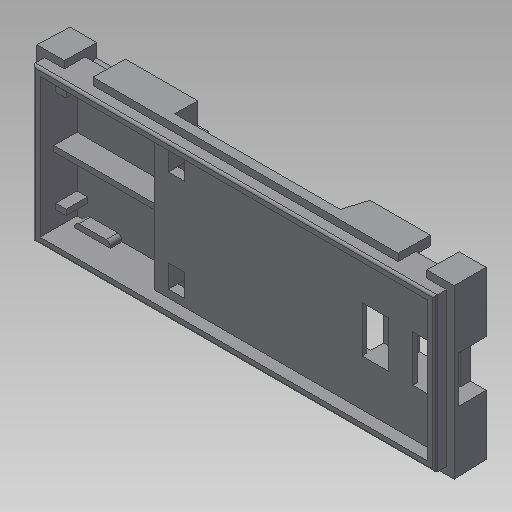
# Autodesk Inventor part: D2MG bottom
Saved by Autodesk Inventor 2018 (Build 220112000, 112)
## iProperties
Created: 2015-02-09
Part Number: D2MG bottom
Material: Типовые
Document SubType Name: Modeling
Designer: Abbath
Density: 1 g/cm^3
Appearance: По умолчанию
Mass: 9.33174 g
Surface Area: 109.957 cm^2
Volume: 9.33174 cm^3
Author: Abbath
Autodesk Inventor part; units mm, degrees
sketch "Эскиз2" plane through (0, 0, 0) normal (0, 1, 0) x (-1, 0, 0)
  line L0 (45.1, 0) -> (-45.1, 0)
  line L1 (-45.1, 0) -> (-44.9342, -9.5)
  line L2 (-44.9342, -9.5) -> (44.9342, -9.5)
  line L3 (44.9342, -9.5) -> (45.1, 0)
  line L4 (-45.1, 0) -> (-45.1, -33.7167) construction
  line L5 (45.1, 0) -> (45.1, -29.7578) construction
  point P0 (0, 0)
  point P1 (0, 0)
  dimension "d4" = 9.5
  dimension "d5" = 90.2
  dimension "d6" = 1
  dimension "d7" = 1
  constraints: 12 end point, 2 vertical, 1 coincident, 1 horizontal, 1 midpoint, 1 parallel
  measures "d4" distance between parallel lines of L2 L0
  measures "d5" distance of L0.start L0.end
  measures "d6" angle of L4 L1
  measures "d7" angle of L3 L5
sketch "Эскиз3" plane through (0, 0, 0) normal (1, 0, 0) x (0, 1, 0)
  line L0 (-18.15, 0) -> (18.15, 0)
  line L1 (18.15, 0) -> (17.9842, -9.5)
  line L2 (17.9842, -9.5) -> (-17.9842, -9.5)
  line L3 (-17.9842, -9.5) -> (-18.15, 0)
  line L4 (18.15, 0) -> (18.15, -16.3653) construction
  line L5 (-18.15, 0) -> (-18.15, -16.3653) construction
  point P0 (0, 0)
  point P1 (0, 0)
  point P2 (0, -9.5)
  point P3 (0, 0)
  point P4 (0, -9.5)
  dimension "d8" = 1
  dimension "d9" = 1
  dimension "d10" = 36.3
  constraints: 12 end point, 2 coincident, 2 midpoint, 2 vertical, 1 horizontal, 1 parallel
  measures "d8" angle of L5 L3
  measures "d9" angle of L4 L1
  measures "d10" distance of L0.start L0.end
ref_plane "РабПлоскость1" through (-45.1, 0, 0) normal (0, 0, 1) x (1, 0, 0)
sketch "Эскиз4" plane through (-45.1, 0, 0) normal (0, 0, 1) x (1, 0, 0)
  line L0 (0, 18.15) -> (90.2, 18.15)
  line L1 (90.2, 18.15) -> (90.2, -18.15)
  line L2 (90.2, -18.15) -> (0, -18.15)
  line L3 (0, -18.15) -> (0, 18.15)
  point P0 (45.1, 0)
  point P1 (0, 0)
  point P2 (45.1, 18.15)
  point P3 (90.2, 0)
  point P4 (45.1, -18.15)
  constraints: 8 end point, 4 midpoint, 2 parallel, 1 horizontal, 1 perpendicular
ref_plane "РабПлоскость2" through (44.9342, 0, -9.5) normal (0, 0, 1) x (-1, 0, 0)
sketch "Эскиз5" plane through (44.9342, 0, -9.5) normal (0, 0, 1) x (-1, 0, 0)
  line L0 (89.8684, -17.9842) -> (0, -17.9842)
  line L1 (0, -17.9842) -> (0, 17.9842)
  line L2 (0, 17.9842) -> (89.8684, 17.9842)
  line L3 (89.8684, 17.9842) -> (89.8684, -17.9842)
  point P0 (44.9342, 0)
  point P1 (89.8684, 0)
  point P2 (44.9342, -17.9842)
  point P3 (0, 0)
  point P4 (44.9342, 17.9842)
  constraints: 8 end point, 4 midpoint, 2 parallel, 1 horizontal, 1 perpendicular
loft "Лофт1" add profiles "Эскиз5", "Эскиз4"
sketch "Эскиз6" plane through (-45.1, 18.15, 0) normal (0, 0, 1) x (1, 0, 0)
  line L0 (1.7, -34.7) -> (88.5, -34.7)
  line L1 (88.5, -34.7) -> (88.5, -1.6)
  line L2 (88.5, -1.6) -> (1.7, -1.6)
  line L3 (1.7, -1.6) -> (1.7, -34.7)
  line L4 (0, -36.3) -> (0, 0) construction
  line L5 (90.2, -36.3) -> (0, -36.3) construction
  line L6 (90.2, 0) -> (90.2, -36.3) construction
  line L7 (0, 0) -> (90.2, 0) construction
  line L8 (-1, -37.3) -> (91.2, -37.3)
  line L9 (91.2, -37.3) -> (91.2, 1)
  line L10 (91.2, 1) -> (-1, 1)
  line L11 (-1, 1) -> (-1, -37.3)
  point P0 (45.1, -18.15)
  point P1 (45.1, -1.6)
  point P2 (1.7, -18.15)
  dimension "d21" = 86.8
  dimension "d22" = 1.7
  dimension "d23" = 1.7
  dimension "d24" = 33.1
  dimension "d25" = 1.6
  dimension "d26" = 1.6
  dimension "d27" = 1
  dimension "d28" = 1
  dimension "d29" = 1
  dimension "d30" = 1
  constraints: 16 end point, 4 parallel, 2 horizontal, 2 midpoint, 2 perpendicular, 1 horizontal alignment, 1 vertical alignment
  measures "d21" distance between parallel lines of L1 L3
  measures "d22" distance between parallel lines of L3 L4
  measures "d23" distance between parallel lines of L6 L1
  measures "d24" distance between parallel lines of L2 L0
  measures "d25" distance between parallel lines of L0 L5
  measures "d26" distance between parallel lines of L7 L2
  measures "d27" distance between parallel lines of L4 L11
  measures "d28" distance between parallel lines of L10 L7
  measures "d29" distance between parallel lines of L9 L6
  measures "d30" distance between parallel lines of L8 L5
extrude "Выдавливание2" cut sketch "Эскиз6" against normal blind 2.5
sketch "Эскиз7" plane through (-43.4, 16.55, 0) normal (0, 0, 1) x (1, 0, 0)
  line L0 (1.5, -31.6) -> (85.3, -31.6)
  line L1 (85.3, -31.6) -> (85.3, -1.5)
  line L2 (85.3, -1.5) -> (1.5, -1.5)
  line L3 (1.5, -1.5) -> (1.5, -31.6)
  line L4 (86.8, -33.1) -> (86.8, 0) construction
  line L5 (86.8, 0) -> (0, 0) construction
  line L6 (0, 0) -> (0, -33.1) construction
  line L7 (0, -33.1) -> (86.8, -33.1) construction
  point P0 (43.4, -16.55)
  dimension "d33" = 1.5
  dimension "d34" = 1.5
  dimension "d35" = 1.5
  dimension "d36" = 1.5
  constraints: 8 end point, 2 parallel, 1 horizontal, 1 perpendicular
  measures "d33" distance between parallel lines of L3 L6
  measures "d34" distance between parallel lines of L2 L5
  measures "d35" distance between parallel lines of L1 L4
  measures "d36" distance between parallel lines of L0 L7
extrude "Выдавливание3" cut sketch "Эскиз7" against normal blind 2.5
sketch "Эскиз8" plane through (-43.4, 16.55, -2.5) normal (0, 0, 1) x (1, 0, 0)
  line L0 (1.5, -1.5) -> (23.8, -1.5)
  line L1 (23.8, -1.5) -> (23.8, -31.6)
  line L2 (23.8, -31.6) -> (1.5, -31.6)
  line L3 (1.5, -31.6) -> (1.5, -1.5)
  line L4 (85.3, -31.6) -> (1.5, -31.6) construction
  line L5 (85.3, -1.5) -> (85.3, -31.6) construction
  line L6 (1.5, -1.5) -> (85.3, -1.5) construction
  line L7 (1.5, -31.6) -> (1.5, -1.5) construction
  point P0 (43.4, -16.55)
  dimension "d39" = 22.3
  constraints: 8 end point, 3 collinear, 2 parallel, 1 horizontal, 1 perpendicular
  measures "d39" distance between parallel lines of L1 L3
extrude "Выдавливание4" cut sketch "Эскиз8" against normal blind 5.5
sketch "Эскиз9" plane through (0, 0, 0) normal (0, 1, 0) x (-1, 0, 0)
  line L0 (19.6, -8) -> (41.9, -8)
  line L1 (41.9, -8) -> (41.9, -3)
  line L2 (41.9, -3) -> (19.6, -3)
  line L3 (19.6, -3) -> (19.6, -8)
  line L4 (19.6, -2.5) -> (19.6, -8) construction
  line L5 (19.6, -8) -> (41.9, -8) construction
  line L6 (41.9, 0) -> (41.9, -8) construction
  line L7 (-44.9342, -9.5) -> (44.9342, -9.5) construction
  line L8 (-41.9, -2.5) -> (19.6, -2.5) construction
  point P0 (0, 0)
  dimension "d43" = 0.5
  constraints: 8 end point, 3 collinear, 2 parallel, 1 horizontal, 1 perpendicular
  measures "d43" distance between parallel lines of L2 L8
extrude "Выдавливание5" add sketch "Эскиз9" along normal mid plane 1.2
sketch "Эскиз10" plane through (-43.4, 16.55, 0) normal (0, 0, 1) x (1, 0, 0)
  line L0 (4.25, -33.1) -> (10.45, -33.1)
  line L1 (10.45, -33.1) -> (10.45, -35.6564)
  line L2 (10.45, -35.6564) -> (4.25, -35.6564)
  line L3 (4.25, -35.6564) -> (4.25, -33.1)
  line L4 (4.25, 2.5564) -> (10.45, 2.5564)
  line L5 (10.45, 2.5564) -> (10.45, 0)
  line L6 (10.45, 0) -> (4.25, 0)
  line L7 (4.25, 0) -> (4.25, 2.5564)
  line L8 (76.35, 0) -> (82.55, 0)
  line L9 (82.55, 0) -> (82.55, 2.5564)
  line L10 (82.55, 2.5564) -> (76.35, 2.5564)
  line L11 (76.35, 2.5564) -> (76.35, 0)
  line L12 (76.35, -33.1) -> (82.55, -33.1)
  line L13 (82.55, -33.1) -> (82.55, -35.6564)
  line L14 (82.55, -35.6564) -> (76.35, -35.6564)
  line L15 (76.35, -35.6564) -> (76.35, -33.1)
  line L16 (7.35, -51.2865) -> (7.35, 35.2838) construction
  line L17 (79.45, -51.2865) -> (79.45, 29.244) construction
  line L18 (-1.6564, 1.5564) -> (88.4564, 1.5564) construction
  line L19 (-1.6564, -34.6564) -> (-1.6564, 1.5564) construction
  line L20 (88.4564, -34.6564) -> (-1.6564, -34.6564) construction
  line L21 (88.4564, 1.5564) -> (88.4564, -34.6564) construction
  line L22 (86.8, -33.1) -> (86.8, 0) construction
  line L23 (0, -33.1) -> (86.8, -33.1) construction
  line L24 (0, 0) -> (0, -33.1) construction
  line L25 (86.8, 0) -> (0, 0) construction
  line L26 (86.8, 0) -> (0, 0) construction
  point P0 (43.4, -16.55)
  point P1 (7.35, 2.5564)
  point P2 (7.35, -35.6564)
  point P3 (79.45, -35.6564)
  point P4 (79.45, 0)
  dimension "d46" = 72.1
  dimension "d47" = 36.05
  dimension "d48" = 6.2
  dimension "d49" = 1
  constraints: 36 end point, 8 parallel, 6 point on line, 5 collinear, 4 horizontal, 4 midpoint, 4 perpendicular, 3 equal length, 2 vertical
  measures "d46" distance between parallel lines of L17 L16
  measures "d47" distance from line of point (43.4, -16.55) L16
  measures "d48" distance between parallel lines of L5 L7
  measures "d49" distance between parallel lines of L10 L18
extrude "Выдавливание6" cut sketch "Эскиз10" against normal through all
sketch "Эскиз11" plane through (-43.4, 16.55, -8) normal (0, 0, 1) x (1, 0, 0)
  line L0 (1.5, -31.6) -> (1.5, -1.5) construction
  line L1 (85.3, -31.6) -> (1.5, -31.6) construction
  line L2 (1.5, -1.5) -> (85.3, -1.5) construction
  line L3 (3.5, -31.6) -> (11.2, -31.6)
  line L4 (3.5, -31.6) -> (3.5, -31.3)
  line L5 (4.4, -30.4) -> (10.3, -30.4)
  line L6 (11.2, -31.3) -> (11.2, -31.6)
  line L7 (3.5, -1.5) -> (11.2, -1.5)
  line L8 (11.2, -1.5) -> (11.2, -1.8)
  line L9 (10.3, -2.7) -> (4.4, -2.7)
  line L10 (3.5, -1.8) -> (3.5, -1.5)
  arc A0 (3.5, -1.8) -> (4.4, -2.7) centre (4.4, -1.8) ccw
  arc A1 (10.3, -2.7) -> (11.2, -1.8) centre (10.3, -1.8) ccw
  arc A2 (4.4, -30.4) -> (3.5, -31.3) centre (4.4, -31.3) ccw
  arc A3 (11.2, -31.3) -> (10.3, -30.4) centre (10.3, -31.3) ccw
  line L11 (1.5, -28.15) -> (3.7436, -28.15)
  line L12 (3.7436, -28.15) -> (3.7436, -26.95)
  line L13 (3.7436, -26.95) -> (1.5, -26.95)
  line L14 (1.5, -26.95) -> (1.5, -28.15)
  line L15 (1.5, -6.15) -> (3.7436, -6.15)
  line L16 (3.7436, -6.15) -> (3.7436, -4.95)
  line L17 (3.7436, -4.95) -> (1.5, -4.95)
  line L18 (1.5, -4.95) -> (1.5, -6.15)
  line L19 (4.25, -33.1) -> (4.25, -34.5342) projected
  line L20 (10.45, -34.5342) -> (10.45, -33.1) projected
  line L21 (-1.6564, -34.6564) -> (-1.6564, 1.5564) projected
  point P0 (43.4, -16.55)
  dimension "d52" = 7.7
  dimension "d53" = 0.75
  dimension "d54" = 0.75
  dimension "d55" = 1.2
  dimension "d56" = 0.9
  dimension "d57" = 20.8
  dimension "d58" = 10.4
  dimension "d59" = 23.2
  dimension "d72" = 5.4
  constraints: 32 end point, 8 point on circle, 8 tangent, 7 perpendicular, 5 collinear, 4 centre point, 4 horizontal, 4 parallel, 3 equal radius, 2 equal length, 2 point on line, 1 vertical
  measures "d52" distance between parallel lines of L6 L4
  measures "d53" distance between parallel lines of L19 L4
  measures "d54" distance between parallel lines of L6 L20
  measures "d55" distance between parallel lines of L5 L3
  measures "d56" radius of A2
  measures "d57" distance between parallel lines of L15 L13
  measures "d58" distance from line of point (43.4, -16.55) L13
  measures "d59" distance between parallel lines of L17 L11
  measures "d72" distance between parallel lines of L16 L21
extrude "Выдавливание7" add sketch "Эскиз11" along normal blind 4.6 contours L14 L13 L12 L11 | L18 L17 L16 L15
fillet "Сопряжение1" radius 0.5 4 edges at (0, -16.55, 0) (43.4, 0, 0) (0, 16.55, 0) (-43.4, 0, 0)
sketch "Эскиз12" plane through (-32.95, -16.55, -2.5) normal (0, -1, 0) x (1, 0, 0)
  line L0 (-6.2, -7) -> (-6.2, 0) construction
  line L1 (0, 0) -> (0, -7) construction
  line L2 (65.9, -7) -> (65.9, 0) construction
  line L3 (72.1, 0) -> (72.1, -7) construction
  line L4 (-6.2, -4.5) -> (0, -4.5)
  line L5 (0, -4.5) -> (0, -8)
  line L6 (0, -8) -> (-6.2, -8)
  line L7 (-6.2, -8) -> (-6.2, -4.5)
  line L8 (65.9, -4.5) -> (72.1, -4.5)
  line L9 (72.1, -4.5) -> (72.1, -8)
  line L10 (72.1, -8) -> (65.9, -8)
  line L11 (65.9, -8) -> (65.9, -4.5)
  line L12 (65.9, 0) -> (0, 0) construction
  line L13 (0, -7) -> (65.9, -7) construction
  point P0 (32.95, 2.5)
  dimension "d64" = 4.5
  dimension "d65" = 1
  constraints: 16 end point, 4 collinear, 4 parallel, 2 horizontal, 2 perpendicular, 2 point on line
  measures "d64" distance between parallel lines of L4 L12
  measures "d65" distance between parallel lines of L6 L13
extrude "Выдавливание8" cut sketch "Эскиз12" against normal up to surface (1.5 mm away)
sketch "Эскиз13" plane through (-32.95, 16.55, -2.5) normal (0, 1, 0) x (1, 0, 0)
  line L0 (-6.2, 8) -> (-6.2, 4.5) projected
  line L1 (0, 8) -> (-6.2, 8) projected
  line L2 (0, 4.5) -> (0, 8) projected
  line L3 (-6.2, 4.5) -> (0, 4.5) projected
  line L4 (65.9, 4.5) -> (72.1, 4.5) projected
  line L5 (72.1, 4.5) -> (72.1, 8) projected
  line L6 (65.9, 8) -> (65.9, 4.5) projected
  line L7 (72.1, 8) -> (65.9, 8) projected
  point P0 (32.95, -2.5)
extrude "Выдавливание9" cut sketch "Эскиз13" against normal up to surface (1.5 mm away)
extrude "Выдавливание10" add sketch "Эскиз11" along normal blind 2.5 contours L4 A2 L5 A3 L6 L3 | L7 L8 A1 L9 A0 L10
ref_plane "РабПлоскость3" through (-32.95, 0, -2.5) normal (0, -1, 0) x (1, 0, 0)
ref_plane "РабПлоскость4" through (0, -16.55, -2.5) normal (1, 0, 0) x (0, 0, -1)
sketch "Эскиз14" plane through (44.9342, -17.9842, -9.5) normal (0, 0, -1) x (-1, 0, 0)
  line L0 (2, 2) -> (62.2684, 2)
  line L1 (62.2684, 2) -> (62.2684, 33.9684)
  line L2 (62.2684, 33.9684) -> (2, 33.9684)
  line L3 (2, 33.9684) -> (2, 2)
  line L4 (89.8684, 0) -> (89.8684, 35.9684) construction
  line L5 (11.9842, 0) -> (77.8842, 0) construction
  line L6 (77.8842, 35.9684) -> (11.9842, 35.9684) construction
  line L7 (0, 35.9684) -> (0, 0) construction
  line L8 (5.7842, 35.9684) -> (0, 35.9684) projected
  point P0 (44.9342, 17.9842)
  dimension "d73" = 27.6
  dimension "d74" = 2
  dimension "d75" = 2
  dimension "d76" = 2
  constraints: 8 end point, 2 parallel, 1 horizontal, 1 perpendicular
  measures "d73" distance between parallel lines of L1 L4
  measures "d74" distance between parallel lines of L3 L7
  measures "d75" distance between parallel lines of L2 L8
  measures "d76" distance between parallel lines of L0 L5
extrude "Выдавливание11" cut sketch "Эскиз14" against normal blind 5
sketch "Эскиз15" plane through (0, 0, 0) normal (0, 1, 0) x (-1, 0, 0)
  line L0 (17.3342, -9.5) -> (17.3342, -4.5) construction
  line L1 (-42.9342, -4.5) -> (17.3342, -4.5) construction
  line L2 (17.3342, -9.5) -> (17.3342, -4.5)
  line L3 (17.3342, -4.5) -> (-18.4658, -4.5)
  line L4 (-18.4658, -4.5) -> (-19.8658, -9.5)
  line L5 (-19.8658, -9.5) -> (17.3342, -9.5)
  line L6 (-32.95, -9.5) -> (17.3342, -9.5) construction
  point P0 (0, 0)
  dimension "d79" = 35.8
  dimension "d80" = 37.2
  constraints: 8 end point, 3 collinear, 2 horizontal, 1 vertical
  measures "d79" distance from line of L3.end L0
  measures "d80" distance from line of L4.end L0
extrude "Выдавливание12" cut sketch "Эскиз15" along normal through all both and the other way through all
ref_plane "РабПлоскость5" through (44.9342, -17.9842, -3.5) normal (0, 0, -1) x (-1, 0, 0)
sketch "Эскиз16" plane through (44.9342, -17.9842, -3.5) normal (0, 0, -1) x (-1, 0, 0)
  line L0 (0, 35.9684) -> (0, 0) construction
  line L1 (62.2684, 35.9684) -> (62.2684, 0) construction
  line L2 (62.2684, -0.0873) -> (26.4684, -0.0873) construction
  line L3 (26.4684, 36.0556) -> (62.2684, 36.0556) construction
  line L4 (-5, 12.9842) -> (51.9905, 12.9842)
  line L5 (51.9905, 12.9842) -> (51.9905, 22.9842)
  line L6 (51.9905, 22.9842) -> (-5, 22.9842)
  line L7 (-5, 22.9842) -> (-5, 12.9842)
  line L8 (89.9905, -0.1222) -> (89.9905, 36.0905) construction
  point P0 (44.9342, 17.9842)
  point P1 (51.9905, 17.9842)
  dimension "d84" = 10
  dimension "d85" = 5
  dimension "d86" = 38
  constraints: 8 end point, 2 parallel, 1 horizontal, 1 horizontal alignment, 1 midpoint, 1 perpendicular
  measures "d84" distance between parallel lines of L6 L4
  measures "d85" distance between parallel lines of L7 L0
  measures "d86" distance between parallel lines of L5 L8
extrude "Выдавливание13" cut sketch "Эскиз16" along normal through all
sketch "Эскиз17" plane through (44.9342, -17.9842, -3.5) normal (0, 0, -1) x (-1, 0, 0)
  line L0 (-0.1047, 12.9842) -> (-0.1047, 22.9842) construction
  line L1 (-0.1047, 12.9842) -> (51.9905, 12.9842) construction
  line L2 (51.9905, 12.9842) -> (51.9905, 22.9842) construction
  line L3 (51.9905, 22.9842) -> (-0.1047, 22.9842) construction
  line L4 (13.9842, 12.9842) -> (19.7842, 12.9842)
  line L5 (19.7842, 12.9842) -> (19.7842, 22.9842)
  line L6 (19.7842, 22.9842) -> (13.9842, 22.9842)
  line L7 (13.9842, 22.9842) -> (13.9842, 12.9842)
  line L8 (3.0342, 12.9842) -> (8.8342, 12.9842)
  line L9 (8.8342, 12.9842) -> (8.8342, 22.9842)
  line L10 (8.8342, 22.9842) -> (3.0342, 22.9842)
  line L11 (3.0342, 22.9842) -> (3.0342, 12.9842)
  line L12 (3.0342, 33.0342) -> (3.0342, 2.9342) construction
  point P0 (44.9342, 17.9842)
  dimension "d89" = 5.8
  dimension "d90" = 5.15
  constraints: 16 end point, 6 collinear, 4 parallel, 2 horizontal, 2 perpendicular
  measures "d89" distance between parallel lines of L9 L12
  measures "d90" distance between parallel lines of L7 L9
extrude "Выдавливание14" cut sketch "Эскиз17" against normal through all
sketch "Эскиз18" plane through (0, 0, 0) normal (0, 1, 0) x (-1, 0, 0)
  line L0 (-32.95, -9.5) -> (-32.95, -2.5) construction
  line L1 (-39.15, -2.5) -> (-39.15, -9.5) construction
  line L2 (-42.9, 0) -> (42.9, 0) construction
  line L3 (-32.95, -6.3) -> (-39.15, -6.3)
  line L4 (-39.15, -6.3) -> (-39.15, -8)
  line L5 (-39.15, -8) -> (-32.95, -8)
  line L6 (-32.95, -8) -> (-32.95, -6.3)
  line L7 (-39.15, -7) -> (-32.95, -7) projected
  point P0 (0, 0)
  dimension "d93" = 1
  dimension "d94" = 6.3
  constraints: 8 end point, 2 collinear, 2 parallel, 1 horizontal, 1 perpendicular
  measures "d93" distance between parallel lines of L5 L7
  measures "d94" distance between parallel lines of L2 L3
extrude "Выдавливание15" cut sketch "Эскиз18" along normal through all both and the other way through all
sketch "Эскиз19" plane through (44.9342, -17.9842, -4.5) normal (0, 0, -1) x (-1, 0, 0)
  line L0 (11.9842, 1.4342) -> (5.7842, 1.4342) construction
  line L1 (5.7842, 34.5342) -> (11.9842, 34.5342) construction
  line L2 (4.4842, 1.4342) -> (13.2842, 1.4342)
  arc A0 (13.2842, 1.4342) -> (11.9842, 2.7342) centre (11.9842, 1.4342) ccw
  line L3 (11.9842, 2.7342) -> (5.7842, 2.7342)
  arc A1 (5.7842, 2.7342) -> (4.4842, 1.4342) centre (5.7842, 1.4342) ccw
  line L4 (4.4842, 34.5342) -> (13.2842, 34.5342)
  arc A2 (11.9842, 33.2342) -> (13.2842, 34.5342) centre (11.9842, 34.5342) ccw
  line L5 (11.9842, 33.2342) -> (5.7842, 33.2342)
  arc A3 (4.4842, 34.5342) -> (5.7842, 33.2342) centre (5.7842, 34.5342) ccw
  line L6 (5.7842, 36.0905) -> (5.7842, 34.5342) construction
  line L7 (11.9842, 34.5342) -> (11.9842, 36.0905) construction
  line L8 (5.7842, 1.4342) -> (5.7842, -0.1222) construction
  line L9 (11.9842, -0.1222) -> (11.9842, 1.4342) construction
  point P0 (44.9342, 17.9842)
  dimension "d97" = 1.3
  dimension "d98" = 1.3
  constraints: 8 end point, 8 point on circle, 8 point on line, 4 centre point, 4 horizontal, 4 vertical alignment, 2 collinear
  measures "d97" distance between parallel lines of L3 L2
  measures "d98" distance between parallel lines of L5 L4
extrude "Выдавливание16" add sketch "Эскиз19" along normal up to surface (1.8 mm away)
sketch "Эскиз20" plane through (44.9342, -17.9842, -4.5) normal (0, 0, -1) x (-1, 0, 0)
  line L0 (19.8778, 24.9842) -> (2, 24.9842)
  line L1 (2, 24.9842) -> (2, 22.9842)
  line L2 (2, 22.9842) -> (19.8778, 22.9842)
  line L3 (19.8778, 22.9842) -> (19.8778, 24.9842)
  line L4 (19.8778, 12.9842) -> (2, 12.9842)
  line L5 (2, 12.9842) -> (2, 10.9842)
  line L6 (2, 10.9842) -> (19.8778, 10.9842)
  line L7 (19.8778, 10.9842) -> (19.8778, 12.9842)
  line L8 (51.9905, 12.9842) -> (2, 12.9842) construction
  line L9 (2, 22.9842) -> (51.9905, 22.9842) construction
  line L10 (2, 22.9842) -> (2, 33.9684) construction
  line L11 (2, 2) -> (2, 12.9842) construction
  line L12 (-0.1222, 36.0905) -> (-0.1222, -0.1222) construction
  point P0 (44.9342, 17.9842)
  dimension "d101" = 14
  dimension "d102" = 20
  constraints: 16 end point, 6 collinear, 4 parallel, 2 horizontal, 2 perpendicular
  measures "d101" distance between parallel lines of L6 L0
  measures "d102" distance between parallel lines of L7 L12
extrude "Выдавливание17" add sketch "Эскиз20" along normal up to surface (5 mm away)
sketch "Эскиз21" plane through (0, 0, 0) normal (0, 1, 0) x (-1, 0, 0)
  line L0 (-44.9342, -9.5) -> (-45.0389, -3.5) construction
  line L1 (-25.0564, -9.5) -> (-44.9342, -9.5) construction
  line L2 (-25.0564, -4.5) -> (-25.0564, -9.5) construction
  line L3 (-25.0564, -7.3) -> (-30.5564, -7.3)
  line L4 (-30.5564, -7.3) -> (-30.5564, -9.5)
  line L5 (-30.5564, -9.5) -> (-25.0564, -9.5)
  line L6 (-25.0564, -9.5) -> (-25.0564, -7.3)
  line L7 (-36.4564, -7.3) -> (-41.5564, -7.3)
  line L8 (-41.5564, -7.3) -> (-41.5564, -9.5)
  line L9 (-41.5564, -9.5) -> (-36.4564, -9.5)
  line L10 (-36.4564, -9.5) -> (-36.4564, -7.3)
  point P0 (0, 0)
  dimension "d105" = 5.5
  dimension "d106" = 5.9
  dimension "d107" = 5.1
  dimension "d108" = 2.2
  constraints: 16 end point, 4 collinear, 4 parallel, 2 horizontal, 2 perpendicular
  measures "d105" distance between parallel lines of L4 L2
  measures "d106" distance between parallel lines of L10 L4
  measures "d107" distance between parallel lines of L8 L10
  measures "d108" distance between parallel lines of L3 L1
extrude "Выдавливание18" add sketch "Эскиз21" along normal up to surface (10 mm away) from surface at -5
sketch "Эскиз22" plane through (44.9342, -17.9842, -4.5) normal (0, 0, -1) x (-1, 0, 0)
  arc A0 (21.1278, 5.7778) -> (21.1278, 3.2778) centre (21.1278, 4.5278) ccw
  arc A1 (22.0278, 3.2778) -> (22.0278, 5.7778) centre (22.0278, 4.5278) ccw
  arc A2 (21.1278, 32.6905) -> (21.1278, 30.1905) centre (21.1278, 31.4405) ccw
  arc A3 (22.0278, 30.1905) -> (22.0278, 32.6905) centre (22.0278, 31.4405) ccw
  line L0 (21.1278, 3.2778) -> (22.0278, 3.2778)
  line L1 (21.1278, 5.7778) -> (22.0278, 5.7778)
  line L2 (21.1278, 30.1905) -> (22.0278, 30.1905)
  line L3 (21.1278, 32.6905) -> (22.0278, 32.6905)
  line L4 (19.8778, 3.5894) -> (19.8778, 6.2353) construction
  line L5 (23.2778, 3.5894) -> (23.2778, 5.4774) construction
  line L6 (11.9842, -0.1222) -> (77.8842, -0.1222) construction
  line L7 (77.8842, 36.0905) -> (11.9842, 36.0905) construction
  line L8 (-0.1222, 36.0905) -> (-0.1222, -0.1222) construction
  point P0 (44.9342, 17.9842)
  dimension "d111" = 3.4
  dimension "d112" = 2.5
  dimension "d113" = 5.9
  dimension "d114" = 5.9
  dimension "d115" = 23.4
  constraints: 12 end point, 10 tangent, 8 point on circle, 4 centre point, 4 horizontal, 2 vertical, 1 equal radius, 1 parallel, 1 vertical alignment
  measures "d111" distance between parallel lines of L5 L4
  measures "d112" distance between parallel lines of L1 L0
  measures "d113" distance between parallel lines of L2 L7
  measures "d114" distance between parallel lines of L1 L6
  measures "d115" distance between parallel lines of L5 L8
extrude "Выдавливание19" add sketch "Эскиз22" along normal blind 3
sketch "Эскиз23" plane through (44.9342, -17.9842, -4.5) normal (0, 0, -1) x (-1, 0, 0)
  line L0 (89.9905, -0.1222) -> (89.9905, 36.0905) construction
  line L1 (77.8842, 36.0905) -> (11.9842, 36.0905) construction
  line L2 (11.9842, -0.1222) -> (77.8842, -0.1222) construction
  line L3 (58.0905, 4.5778) -> (61.5905, 4.5778)
  line L4 (61.5905, 4.5778) -> (61.5905, 9.4842)
  line L5 (61.5905, 9.4842) -> (58.0905, 9.4842)
  line L6 (58.0905, 9.4842) -> (58.0905, 4.5778)
  line L7 (58.0905, 26.4842) -> (61.5905, 26.4842)
  line L8 (61.5905, 26.4842) -> (61.5905, 31.3905)
  line L9 (61.5905, 31.3905) -> (58.0905, 31.3905)
  line L10 (58.0905, 31.3905) -> (58.0905, 26.4842)
  point P0 (44.9342, 17.9842)
  dimension "d118" = 28.4
  dimension "d119" = 4.7
  dimension "d120" = 4.7
  dimension "d121" = 17
  dimension "d122" = 3.5
  constraints: 16 end point, 4 parallel, 3 collinear, 2 horizontal, 2 perpendicular
  measures "d118" distance between parallel lines of L8 L0
  measures "d119" distance between parallel lines of L9 L1
  measures "d120" distance between parallel lines of L3 L2
  measures "d121" distance between parallel lines of L7 L5
  measures "d122" distance between parallel lines of L4 L6
extrude "Выдавливание20" cut sketch "Эскиз23" against normal through all
ref_plane "РабПлоскость6" through (-16.6564, -10.9532, -4.5) normal (0, -1, 0) x (1, 0, 0)
sketch "Эскиз24" plane through (-16.6564, -10.9532, -4.5) normal (0, -1, 0) x (1, 0, 0)
  line L0 (0, 0) -> (-0.6778, 0)
  line L1 (-0.6778, 0) -> (-0.6778, -5)
  line L2 (-0.6778, -5) -> (1.6, -5)
  line L3 (1.6, -5) -> (1.6, -3)
  line L4 (1.6, -3) -> (0, -2.0762)
  line L5 (0, -2.0762) -> (0, 0)
  line L6 (35.1222, 0) -> (-0.6778, 0) construction
  line L7 (-0.6778, 0) -> (-0.6778, -5) construction
  line L8 (0, 0) -> (0, 2) construction
  line L9 (-16.2936, -5) -> (-0.6778, -5) construction
  line L10 (-28.2778, -5) -> (-28.4, 2) construction
  point P0 (16.6564, 4.5)
  dimension "d125" = 30
  dimension "d126" = 2
  dimension "d127" = 60
  constraints: 12 end point, 4 collinear, 3 vertical, 2 horizontal
  measures "d125" distance from line of L3 L10.end
  measures "d126" distance of L2.end L3.end
  measures "d127" angle of L4 L5
extrude "Выдавливание21" add sketch "Эскиз24" along normal up to surface (4.9064 mm away) from surface at -2.4532
ref_plane "РабПлоскость7" through (-16.6564, 10.9532, -4.5) normal (0, 1, 0) x (1, 0, 0)
sketch "Эскиз25" plane through (-16.6564, 10.9532, -4.5) normal (0, 1, 0) x (1, 0, 0)
  line L0 (0, 0) -> (0, 2.0762) projected
  line L1 (-0.6778, 0) -> (0, 0) projected
  line L2 (-0.6778, 5) -> (-0.6778, 0) projected
  line L3 (1.6, 5) -> (-0.6778, 5) projected
  line L4 (1.6, 3) -> (1.6, 5) projected
  line L5 (0, 2.0762) -> (1.6, 3) projected
  point P0 (16.6564, -4.5)
extrude "Выдавливание22" add sketch "Эскиз25" against normal up to surface (4.9064 mm away) from surface at 2.4532
sketch "Эскиз26" plane through (44.9342, -17.9842, -4.5) normal (0, 0, -1) x (-1, 0, 0)
  arc A0 (58.0905, 12.9842) -> (59.9905, 12.9842) centre (59.0405, 12.9842) ccw
  arc A1 (59.9905, 22.9842) -> (58.0905, 22.9842) centre (59.0405, 22.9842) ccw
  line L0 (58.0905, 12.9842) -> (58.0905, 22.9842)
  line L1 (59.9905, 12.9842) -> (59.9905, 22.9842)
  line L2 (58.0905, 4.5778) -> (58.0905, 9.4842) projected
  line L3 (59.9905, 31.3905) -> (59.9905, 26.4842) projected
  point P0 (44.9342, 17.9842)
  point P1 (51.9905, 12.9842)
  point P2 (51.9905, 22.9842)
  point P3 (59.9905, 17.9842)
  point P4 (59.9905, 28.9374)
  constraints: 4 end point, 4 point on circle, 4 tangent, 2 centre point, 2 horizontal alignment, 2 midpoint, 2 vertical, 1 collinear, 1 vertical alignment
extrude "Выдавливание23" add sketch "Эскиз26" along normal blind 0.5
equation "\"d47\" = 0.5 * d46"
equation "\"d53\" = d54"
equation "\"d58\" = 0.5 * d57"
equation "\"d98\" = d97"
equation "\"d114\" = d113"
equation "\"d120\" = d119"
